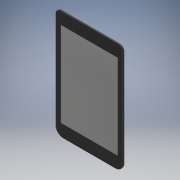
# Autodesk Inventor part: Touchcreen+Cover
Saved by Autodesk Inventor 2017 (Build 210142000, 142)
## iProperties
Created: 2018-08-06
Part Number: Touchcreen+Cover
Material: Generic
Document SubType Name: Modeling
Designer: intelsath
Density: 1 g/cm^3
Appearance: Default
Author: intelsath
Autodesk Inventor part; units mm, degrees
ref_plane "YZ Plane" through (0, 0, 0) normal (1, 0, 0) x (0, 1, 0)
sketch "Sketch2" plane through (0, 0, 0) normal (0, 1, 0) x (-1, 0, 0)
  line L0 (-25.3, 47.42) -> (25.3, 47.42)
  line L1 (29.3, 43.42) -> (29.3, -40.92)
  line L2 (22.8, -47.42) -> (-22.8, -47.42)
  line L3 (-29.3, -40.92) -> (-29.3, 43.42)
  arc A0 (-25.3, 47.42) -> (-29.3, 43.42) centre (-25.3, 43.42) ccw
  arc A1 (29.3, 43.42) -> (25.3, 47.42) centre (25.3, 43.42) ccw
  arc A2 (22.8, -47.42) -> (29.3, -40.92) centre (22.8, -40.92) ccw
  arc A3 (-29.3, -40.92) -> (-22.8, -47.42) centre (-22.8, -40.92) ccw
  point P0 (0, 0)
  point P1 (-29.3, 47.42)
  point P2 (29.3, -47.42)
  point P3 (29.3, 47.42)
  dimension "d6" = 94.84
  dimension "d7" = 58.6
  dimension "d8" = 29.3
  dimension "d9" = 47.42
  dimension "d23" = 4
  dimension "d24" = 4
  dimension "d25" = 6.5
  dimension "d26" = 6.5
  constraints: 8 end point, 8 point on circle, 8 tangent, 6 point on line, 4 centre point, 2 parallel, 1 horizontal, 1 perpendicular
  measures "d6" distance of point (29.3, 47.42) point (29.3, -47.42)
  measures "d7" distance of point (-29.3, 47.42) point (29.3, 47.42)
  measures "d8" distance from line of point (0, 0) L3
  measures "d9" distance from line of point (0, 0) L0
  measures "d23" radius of A0
  measures "d24" radius of A1
  measures "d25" radius of A3
  measures "d26" radius of A2
extrude "Extrusion2" add sketch "Sketch2" along normal blind 1.125
sketch "Sketch1" plane through (0, 0, 0) normal (0, 1, 0) x (-1, 0, 0)
  line L0 (24.78, 37.02) -> (-24.78, 37.02)
  line L1 (-24.78, 37.02) -> (-24.78, -37.02)
  line L2 (-24.78, -37.02) -> (24.78, -37.02)
  line L3 (24.78, -37.02) -> (24.78, 37.02)
  point P0 (0, 0)
  dimension "d0" = 49.56
  dimension "d1" = 74.04
  dimension "d2" = 37.02
  dimension "d3" = 24.78
  constraints: 8 end point, 2 parallel, 1 horizontal, 1 perpendicular
  measures "d0" distance of L1.end L2.end
  measures "d1" distance of L0.end L1.end
  measures "d2" distance from line of L2 point (0, 0)
  measures "d3" distance from line of L1 point (0, 0)
extrude "Extrusion1" cut sketch "Sketch1" along normal blind 1.3
ref_plane "Work Plane1" through (0, 0.02, 0) normal (0, -1, 0) x (1, 0, 0)
ref_plane "Work Plane2" through (0, 1.105, 0) normal (0, 1, 0) x (1, 0, 0)
sketch "Sketch4" plane through (0, 1.105, 0) normal (0, 1, 0) x (1, 0, 0)
  line L0 (-24.78, -37.02) -> (-24.78, 37.02) projected
  line L1 (24.78, -37.02) -> (-24.78, -37.02) projected
  line L2 (24.78, 37.02) -> (24.78, -37.02) projected
  line L3 (-24.78, 37.02) -> (24.78, 37.02) projected
  line L4 (-24.78, -37.02) -> (-24.78, 37.02) projected
  line L5 (-24.78, 37.02) -> (24.78, 37.02) projected
  line L6 (24.78, 37.02) -> (24.78, -37.02) projected
  line L7 (24.78, -37.02) -> (-24.78, -37.02) projected
  line L8 (29.3, -43.42) -> (29.3, 40.92) projected
  arc A0 (29.3, 40.92) -> (22.8, 47.42) centre (22.8, 40.92) ccw projected
  line L9 (22.8, 47.42) -> (-22.8, 47.42) projected
  arc A1 (-22.8, 47.42) -> (-29.3, 40.92) centre (-22.8, 40.92) ccw projected
  line L10 (-29.3, 40.92) -> (-29.3, -43.42) projected
  arc A2 (-29.3, -43.42) -> (-25.3, -47.42) centre (-25.3, -43.42) ccw projected
  line L11 (-25.3, -47.42) -> (25.3, -47.42) projected
  arc A3 (25.3, -47.42) -> (29.3, -43.42) centre (25.3, -43.42) ccw projected
  line L12 (-24.78, -37.02) -> (24.78, -37.02) projected
  line L13 (-24.78, -37.02) -> (24.78, -37.02)
  line L14 (24.78, -37.02) -> (24.78, 37.02)
  line L15 (24.78, 37.02) -> (-24.78, 37.02)
  line L16 (-24.78, 37.02) -> (-24.78, -37.02)
  point P0 (0, 0)
  constraints: 8 end point, 2 parallel, 1 horizontal, 1 perpendicular
extrude "Extrusion4" add sketch "Sketch4" along normal up to surface (1.085 mm away) from surface at -1.085 contours L0 L3 L2 L1
equation "\"d8\" = 0.5 * d7"
equation "\"d9\" = 0.5 * d6"
equation "\"d24\" = d23"
equation "\"d26\" = d25"
equation "\"d2\" = 0.5 * d1"
equation "\"d3\" = 0.5 * d0"
body "Solid1"
